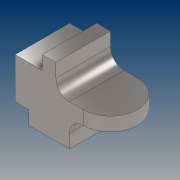
# Autodesk Inventor part: 21
Saved by Autodesk Inventor 2020.2 (Build 242310000, 310)
## iProperties
Created: 2020-09-17
Part Number: 21
Material: 鋼、碳鋼
Document SubType Name: Modeling
Designer: user
Density: 7.85 g/cm^3
Appearance: 半拋光
Mass: 565.2 g
Surface Area: 124.274 cm^2
Volume: 72 cm^3
Author: user
Autodesk Inventor part; units mm, degrees
ref_plane "YZ Plane" through (0, 0, 0) normal (1, 0, 0) x (0, 1, 0)
ref_plane "XZ Plane" through (0, 0, 0) normal (0, 1, 0) x (-1, 0, 0)
ref_plane "XY Plane" through (0, 0, 0) normal (0, 0, 1) x (1, 0, 0)
sketch "草圖1" plane through (0, 0, 0) normal (0, 0, 1) x (1, 0, 0)
  line L0 (0, 0) -> (0, 40)
  line L1 (0, 40) -> (20, 40)
  line L2 (20, 40) -> (20, 50)
  line L3 (20, 50) -> (30, 50)
  line L4 (30, 50) -> (30, 40)
  arc A0 (30, 40) -> (40, 30) centre (40, 40) ccw
  line L5 (40, 30) -> (70, 30)
  line L6 (70, 30) -> (70, 20)
  line L7 (70, 20) -> (50, 20)
  arc A1 (50, 20) -> (40, 10) centre (50, 10) ccw
  line L8 (40, 10) -> (40, 0)
  line L9 (40, 0) -> (0, 0)
  line L10 (0, 0) -> (10, 0)
  line L11 (10, 0) -> (10, 10)
  line L12 (10, 10) -> (0, 10)
  line L13 (0, 10) -> (0, 0)
  dimension "d0" = 40
  dimension "d1" = 20
  dimension "d2" = 10
  dimension "d3" = 50
  dimension "d4" = 70
  dimension "d5" = 40
  dimension "d6" = 10
  dimension "d7" = 20
  dimension "d8" = 10
  dimension "d9" = 10
  dimension "d10" = 10
  constraints: 28 end point, 11 perpendicular, 4 point on circle, 4 tangent, 2 centre point, 2 parallel, 1 horizontal, 1 vertical
  measures "d0" distance between parallel lines of L1 L9
  measures "d1" distance of L0.end L1.end
  measures "d2" distance of L2.end L3.end
  measures "d3" distance between parallel lines of L3 L9
  measures "d4" distance between parallel lines of L6 L0
  measures "d5" distance between parallel lines of L8 L0
  measures "d6" distance of L5.end L6.end
  measures "d7" distance between parallel lines of L7 L9
  measures "d8" radius of A1
  measures "d9" radius of A0
  measures "d10" distance of L10.end L11.end
extrude "擠出1" add sketch "草圖1" along normal mid plane 40 contours L0 L1 L2 L3 L4 A0 L5 L6 L7 A1 L8 L9 L11 L12
fillet "圓角1" radius 20 2 edges at (70, 25, 20) (70, 25, -20)
